minecraftdiamondsword for big CNC schetch rotated_v3 (Autodesk Fusion 360 design; units mm, degrees)
Autodesk Fusion 360 part; units mm, degrees
sketch "big huge diamond sword" plane through (0, 0, 0) normal (0, 0, 1) x (1, 0, 0)
  line L0 (0, 45.2548) -> (5.6569, 39.598)
  line L1 (5.6569, 39.598) -> (11.3137, 45.2548)
  line L2 (11.3137, 45.2548) -> (5.6569, 50.9117)
  line L3 (5.6569, 50.9117) -> (0, 45.2548)
  line L4 (5.6569, 39.598) -> (11.3137, 33.9411)
  line L5 (11.3137, 33.9411) -> (16.9706, 39.598)
  line L6 (16.9706, 39.598) -> (11.3137, 45.2548)
  line L7 (11.3137, 45.2548) -> (5.6569, 39.598)
  line L8 (11.3137, 33.9411) -> (16.9706, 28.2843)
  line L9 (16.9706, 28.2843) -> (22.6274, 33.9411)
  line L10 (16.9706, 39.598) -> (11.3137, 33.9411)
  line L11 (5.6569, 50.9117) -> (11.3137, 45.2548)
  line L12 (11.3137, 45.2548) -> (16.9706, 50.9117)
  line L13 (16.9706, 50.9117) -> (11.3137, 56.5685)
  line L14 (11.3137, 56.5685) -> (5.6569, 50.9117)
  line L15 (16.9706, 50.9117) -> (22.6274, 45.2548)
  line L16 (22.6274, 45.2548) -> (16.9706, 39.598)
  line L17 (16.9706, 39.598) -> (11.3137, 45.2548)
  line L18 (11.3137, 45.2548) -> (16.9706, 50.9117)
  line L19 (11.3137, 56.5685) -> (16.9706, 50.9117)
  line L20 (16.9706, 50.9117) -> (22.6274, 56.5685)
  line L21 (22.6274, 56.5685) -> (16.9706, 62.2254)
  line L22 (16.9706, 62.2254) -> (11.3137, 56.5685)
  line L23 (16.9706, 50.9117) -> (22.6274, 45.2548)
  line L24 (22.6274, 45.2548) -> (28.2843, 50.9117)
  line L25 (28.2843, 50.9117) -> (22.6274, 56.5685)
  line L26 (22.6274, 56.5685) -> (16.9706, 50.9117)
  line L27 (22.6274, 45.2548) -> (28.2843, 39.598)
  line L28 (28.2843, 39.598) -> (22.6274, 33.9411)
  line L29 (22.6274, 33.9411) -> (16.9706, 39.598)
  line L30 (16.9706, 39.598) -> (22.6274, 45.2548)
  line L31 (22.6274, 45.2548) -> (28.2843, 39.598)
  line L32 (28.2843, 39.598) -> (33.9411, 45.2548)
  line L33 (33.9411, 45.2548) -> (28.2843, 50.9117)
  line L34 (28.2843, 50.9117) -> (22.6274, 45.2548)
  line L35 (28.2843, 50.9117) -> (33.9411, 45.2548)
  line L36 (33.9411, 45.2548) -> (39.598, 50.9117)
  line L37 (39.598, 50.9117) -> (33.9411, 56.5685)
  line L38 (33.9411, 56.5685) -> (28.2843, 50.9117)
  line L39 (33.9411, 45.2548) -> (39.598, 39.598)
  line L40 (39.598, 39.598) -> (33.9411, 33.9411)
  line L41 (33.9411, 33.9411) -> (28.2843, 39.598)
  line L42 (28.2843, 39.598) -> (33.9411, 45.2548)
  line L43 (33.9411, 45.2548) -> (39.598, 39.598)
  line L44 (39.598, 39.598) -> (45.2548, 45.2548)
  line L45 (45.2548, 45.2548) -> (39.598, 50.9117)
  line L46 (39.598, 50.9117) -> (33.9411, 45.2548)
  line L47 (39.598, 50.9117) -> (45.2548, 45.2548)
  line L48 (45.2548, 45.2548) -> (50.9117, 50.9117)
  line L49 (50.9117, 50.9117) -> (45.2548, 56.5685)
  line L50 (45.2548, 56.5685) -> (39.598, 50.9117)
  line L51 (45.2548, 45.2548) -> (50.9117, 39.598)
  line L52 (45.2548, 33.9411) -> (39.598, 39.598)
  line L53 (39.598, 39.598) -> (45.2548, 45.2548)
  line L54 (45.2548, 45.2548) -> (50.9117, 39.598)
  line L55 (50.9117, 39.598) -> (56.5685, 45.2548)
  line L56 (56.5685, 45.2548) -> (50.9117, 50.9117)
  line L57 (50.9117, 50.9117) -> (45.2548, 45.2548)
  line L58 (50.9117, 50.9117) -> (56.5685, 45.2548)
  line L59 (56.5685, 45.2548) -> (62.2254, 50.9117)
  line L60 (62.2254, 50.9117) -> (56.5685, 56.5685)
  line L61 (56.5685, 56.5685) -> (50.9117, 50.9117)
  line L62 (56.5685, 56.5685) -> (50.9117, 62.2254)
  line L63 (50.9117, 62.2254) -> (56.5685, 67.8823)
  line L64 (56.5685, 67.8823) -> (62.2254, 62.2254)
  line L65 (62.2254, 62.2254) -> (56.5685, 56.5685)
  line L66 (56.5685, 67.8823) -> (62.2254, 62.2254)
  line L67 (62.2254, 62.2254) -> (67.8823, 67.8823)
  line L68 (67.8823, 67.8823) -> (62.2254, 73.5391)
  line L69 (62.2254, 73.5391) -> (56.5685, 67.8823)
  line L70 (62.2254, 73.5391) -> (56.5685, 79.196)
  line L71 (56.5685, 79.196) -> (62.2254, 84.8528)
  line L72 (62.2254, 84.8528) -> (67.8823, 79.196)
  line L73 (67.8823, 79.196) -> (62.2254, 73.5391)
  line L74 (62.2254, 84.8528) -> (67.8823, 79.196)
  line L75 (67.8823, 79.196) -> (73.5391, 84.8528)
  line L76 (73.5391, 84.8528) -> (67.8823, 90.5097)
  line L77 (67.8823, 90.5097) -> (62.2254, 84.8528)
  line L78 (67.8823, 79.196) -> (73.5391, 73.5391)
  line L79 (73.5391, 73.5391) -> (79.196, 79.196)
  line L80 (79.196, 79.196) -> (73.5391, 84.8528)
  line L81 (73.5391, 84.8528) -> (67.8823, 79.196)
  line L82 (62.2254, 73.5391) -> (67.8823, 67.8823)
  line L83 (67.8823, 67.8823) -> (73.5391, 73.5391)
  line L84 (73.5391, 73.5391) -> (67.8823, 79.196)
  line L85 (67.8823, 79.196) -> (62.2254, 73.5391)
  line L86 (73.5391, 73.5391) -> (79.196, 67.8823)
  line L87 (79.196, 67.8823) -> (73.5391, 62.2254)
  line L88 (73.5391, 62.2254) -> (67.8823, 67.8823)
  line L89 (67.8823, 67.8823) -> (73.5391, 73.5391)
  line L90 (67.8823, 67.8823) -> (73.5391, 62.2254)
  line L91 (73.5391, 62.2254) -> (67.8823, 56.5685)
  line L92 (67.8823, 56.5685) -> (62.2254, 62.2254)
  line L93 (62.2254, 62.2254) -> (67.8823, 67.8823)
  line L94 (56.5685, 56.5685) -> (62.2254, 50.9117)
  line L95 (62.2254, 50.9117) -> (67.8823, 56.5685)
  line L96 (67.8823, 56.5685) -> (62.2254, 62.2254)
  line L97 (62.2254, 62.2254) -> (56.5685, 56.5685)
  line L98 (50.9117, 39.598) -> (56.5685, 33.9411)
  line L99 (45.2548, 33.9411) -> (50.9117, 39.598)
  line L100 (56.5685, 45.2548) -> (62.2254, 39.598)
  line L101 (62.2254, 39.598) -> (56.5685, 33.9411)
  line L102 (50.9117, 39.598) -> (56.5685, 45.2548)
  line L103 (62.2254, 50.9117) -> (67.8823, 45.2548)
  line L104 (67.8823, 45.2548) -> (62.2254, 39.598)
  line L105 (62.2254, 39.598) -> (56.5685, 45.2548)
  line L106 (56.5685, 45.2548) -> (62.2254, 50.9117)
  line L107 (56.5685, 33.9411) -> (62.2254, 28.2843)
  line L108 (62.2254, 28.2843) -> (56.5685, 22.6274)
  line L109 (56.5685, 22.6274) -> (50.9117, 28.2843)
  line L110 (50.9117, 28.2843) -> (56.5685, 33.9411)
  line L111 (56.5685, 33.9411) -> (62.2254, 28.2843)
  line L112 (62.2254, 28.2843) -> (67.8823, 33.9411)
  line L113 (67.8823, 33.9411) -> (62.2254, 39.598)
  line L114 (62.2254, 39.598) -> (56.5685, 33.9411)
  line L115 (62.2254, 28.2843) -> (67.8823, 22.6274)
  line L116 (67.8823, 22.6274) -> (62.2254, 16.9706)
  line L117 (62.2254, 16.9706) -> (56.5685, 22.6274)
  line L118 (56.5685, 22.6274) -> (62.2254, 28.2843)
  line L119 (62.2254, 16.9706) -> (67.8823, 11.3137)
  line L120 (67.8823, 11.3137) -> (73.5391, 16.9706)
  line L121 (73.5391, 16.9706) -> (67.8823, 22.6274)
  line L122 (67.8823, 22.6274) -> (62.2254, 16.9706)
  line L123 (67.8823, 11.3137) -> (73.5391, 5.6569)
  line L124 (73.5391, 5.6569) -> (79.196, 11.3137)
  line L125 (79.196, 11.3137) -> (73.5391, 16.9706)
  line L126 (73.5391, 16.9706) -> (67.8823, 11.3137)
  line L127 (62.2254, 16.9706) -> (67.8823, 11.3137)
  line L128 (67.8823, 11.3137) -> (62.2254, 5.6569)
  line L129 (62.2254, 5.6569) -> (56.5685, 11.3137)
  line L130 (56.5685, 11.3137) -> (62.2254, 16.9706)
  line L131 (67.8823, 11.3137) -> (73.5391, 5.6569)
  line L132 (73.5391, 5.6569) -> (67.8823, 0)
  line L133 (67.8823, 0) -> (62.2254, 5.6569)
  line L134 (62.2254, 5.6569) -> (67.8823, 11.3137)
  line L135 (67.8823, 56.5685) -> (73.5391, 50.9117)
  line L136 (73.5391, 50.9117) -> (67.8823, 45.2548)
  line L137 (67.8823, 45.2548) -> (62.2254, 50.9117)
  line L138 (62.2254, 50.9117) -> (67.8823, 56.5685)
  line L139 (67.8823, 45.2548) -> (73.5391, 39.598)
  line L140 (73.5391, 39.598) -> (67.8823, 33.9411)
  line L141 (67.8823, 33.9411) -> (62.2254, 39.598)
  line L142 (62.2254, 39.598) -> (67.8823, 45.2548)
  line L143 (73.5391, 62.2254) -> (79.196, 56.5685)
  line L144 (79.196, 56.5685) -> (73.5391, 50.9117)
  line L145 (73.5391, 50.9117) -> (67.8823, 56.5685)
  line L146 (67.8823, 56.5685) -> (73.5391, 62.2254)
  line L147 (73.5391, 50.9117) -> (79.196, 45.2548)
  line L148 (79.196, 45.2548) -> (73.5391, 39.598)
  line L149 (73.5391, 39.598) -> (67.8823, 45.2548)
  line L150 (67.8823, 45.2548) -> (73.5391, 50.9117)
  line L151 (79.196, 56.5685) -> (84.8528, 50.9117)
  line L152 (84.8528, 50.9117) -> (79.196, 45.2548)
  line L153 (79.196, 45.2548) -> (73.5391, 50.9117)
  line L154 (73.5391, 50.9117) -> (79.196, 56.5685)
  line L155 (67.8823, 33.9411) -> (73.5391, 28.2843)
  line L156 (73.5391, 28.2843) -> (67.8823, 22.6274)
  line L157 (67.8823, 22.6274) -> (62.2254, 28.2843)
  line L158 (62.2254, 28.2843) -> (67.8823, 33.9411)
  line L159 (73.5391, 28.2843) -> (79.196, 22.6274)
  line L160 (79.196, 22.6274) -> (73.5391, 16.9706)
  line L161 (73.5391, 16.9706) -> (67.8823, 22.6274)
  line L162 (67.8823, 22.6274) -> (73.5391, 28.2843)
  line L163 (73.5391, 39.598) -> (79.196, 33.9411)
  line L164 (79.196, 33.9411) -> (73.5391, 28.2843)
  line L165 (73.5391, 28.2843) -> (67.8823, 33.9411)
  line L166 (67.8823, 33.9411) -> (73.5391, 39.598)
  line L167 (79.196, 45.2548) -> (84.8528, 39.598)
  line L168 (84.8528, 39.598) -> (79.196, 33.9411)
  line L169 (79.196, 33.9411) -> (73.5391, 39.598)
  line L170 (73.5391, 39.598) -> (79.196, 45.2548)
  line L171 (79.196, 33.9411) -> (73.5391, 39.598)
  line L172 (73.5391, 39.598) -> (79.196, 45.2548)
  line L173 (79.196, 45.2548) -> (84.8528, 39.598)
  line L174 (84.8528, 39.598) -> (79.196, 33.9411)
  line L175 (79.196, 33.9411) -> (84.8528, 28.2843)
  line L176 (84.8528, 28.2843) -> (90.5097, 33.9411)
  line L177 (90.5097, 33.9411) -> (84.8528, 39.598)
  line L178 (84.8528, 39.598) -> (79.196, 33.9411)
  line L179 (79.196, 45.2548) -> (84.8528, 39.598)
  line L180 (84.8528, 39.598) -> (90.5097, 45.2548)
  line L181 (90.5097, 45.2548) -> (84.8528, 50.9117)
  line L182 (84.8528, 50.9117) -> (79.196, 45.2548)
  line L183 (84.8528, 39.598) -> (90.5097, 33.9411)
  line L184 (90.5097, 33.9411) -> (96.1665, 39.598)
  line L185 (96.1665, 39.598) -> (90.5097, 45.2548)
  line L186 (90.5097, 45.2548) -> (84.8528, 39.598)
  line L187 (90.5097, 33.9411) -> (96.1665, 28.2843)
  line L188 (96.1665, 28.2843) -> (101.8234, 33.9411)
  line L189 (101.8234, 33.9411) -> (96.1665, 39.598)
  line L190 (96.1665, 39.598) -> (90.5097, 33.9411)
  line L191 (79.196, 56.5685) -> (84.8528, 50.9117)
  line L192 (84.8528, 50.9117) -> (90.5097, 56.5685)
  line L193 (90.5097, 56.5685) -> (84.8528, 62.2254)
  line L194 (84.8528, 62.2254) -> (79.196, 56.5685)
  line L195 (84.8528, 50.9117) -> (90.5097, 45.2548)
  line L196 (90.5097, 45.2548) -> (96.1665, 50.9117)
  line L197 (96.1665, 50.9117) -> (90.5097, 56.5685)
  line L198 (90.5097, 56.5685) -> (84.8528, 50.9117)
  line L199 (96.1665, 50.9117) -> (90.5097, 56.5685)
  line L200 (90.5097, 56.5685) -> (96.1665, 62.2254)
  line L201 (96.1665, 62.2254) -> (101.8234, 56.5685)
  line L202 (101.8234, 56.5685) -> (96.1665, 50.9117)
  line L203 (90.5097, 45.2548) -> (96.1665, 39.598)
  line L204 (96.1665, 39.598) -> (101.8234, 45.2548)
  line L205 (101.8234, 45.2548) -> (96.1665, 50.9117)
  line L206 (96.1665, 50.9117) -> (90.5097, 45.2548)
  line L207 (96.1665, 50.9117) -> (101.8234, 45.2548)
  line L208 (101.8234, 45.2548) -> (107.4802, 50.9117)
  line L209 (107.4802, 50.9117) -> (101.8234, 56.5685)
  line L210 (101.8234, 56.5685) -> (96.1665, 50.9117)
  line L211 (96.1665, 39.598) -> (101.8234, 33.9411)
  line L212 (101.8234, 33.9411) -> (107.4802, 39.598)
  line L213 (107.4802, 39.598) -> (101.8234, 45.2548)
  line L214 (101.8234, 45.2548) -> (96.1665, 39.598)
  line L215 (101.8234, 56.5685) -> (107.4802, 50.9117)
  line L216 (107.4802, 50.9117) -> (113.1371, 56.5685)
  line L217 (113.1371, 56.5685) -> (107.4802, 62.2254)
  line L218 (107.4802, 62.2254) -> (101.8234, 56.5685)
  line L219 (101.8234, 33.9411) -> (107.4802, 28.2843)
  line L220 (107.4802, 28.2843) -> (113.1371, 33.9411)
  line L221 (113.1371, 33.9411) -> (107.4802, 39.598)
  line L222 (107.4802, 39.598) -> (101.8234, 33.9411)
  line L223 (101.8234, 45.2548) -> (107.4802, 39.598)
  line L224 (107.4802, 39.598) -> (113.1371, 45.2548)
  line L225 (113.1371, 45.2548) -> (107.4802, 50.9117)
  line L226 (107.4802, 50.9117) -> (101.8234, 45.2548)
  line L227 (113.1371, 45.2548) -> (118.7939, 39.598)
  line L228 (118.7939, 39.598) -> (124.4508, 45.2548)
  line L229 (124.4508, 45.2548) -> (118.7939, 50.9117)
  line L230 (118.7939, 50.9117) -> (113.1371, 45.2548)
  line L231 (113.1371, 45.2548) -> (107.4802, 50.9117)
  line L232 (107.4802, 50.9117) -> (113.1371, 56.5685)
  line L233 (113.1371, 56.5685) -> (118.7939, 50.9117)
  line L234 (118.7939, 50.9117) -> (113.1371, 45.2548)
  line L235 (113.1371, 45.2548) -> (118.7939, 39.598)
  line L236 (118.7939, 39.598) -> (113.1371, 33.9411)
  line L237 (113.1371, 33.9411) -> (107.4802, 39.598)
  line L238 (107.4802, 39.598) -> (113.1371, 45.2548)
  line L239 (113.1371, 56.5685) -> (118.7939, 50.9117)
  line L240 (118.7939, 50.9117) -> (124.4508, 56.5685)
  line L241 (124.4508, 56.5685) -> (118.7939, 62.2254)
  line L242 (118.7939, 62.2254) -> (113.1371, 56.5685)
  line L243 (118.7939, 50.9117) -> (124.4508, 45.2548)
  line L244 (124.4508, 45.2548) -> (130.1076, 50.9117)
  line L245 (130.1076, 50.9117) -> (124.4508, 56.5685)
  line L246 (124.4508, 56.5685) -> (118.7939, 50.9117)
  line L247 (113.1371, 33.9411) -> (118.7939, 28.2843)
  line L248 (118.7939, 28.2843) -> (124.4508, 33.9411)
  line L249 (124.4508, 33.9411) -> (118.7939, 39.598)
  line L250 (118.7939, 39.598) -> (113.1371, 33.9411)
  line L251 (118.7939, 39.598) -> (124.4508, 33.9411)
  line L252 (124.4508, 33.9411) -> (130.1076, 39.598)
  line L253 (130.1076, 39.598) -> (124.4508, 45.2548)
  line L254 (124.4508, 45.2548) -> (118.7939, 39.598)
  line L255 (124.4508, 45.2548) -> (130.1076, 39.598)
  line L256 (130.1076, 39.598) -> (135.7645, 45.2548)
  line L257 (135.7645, 45.2548) -> (130.1076, 50.9117)
  line L258 (130.1076, 50.9117) -> (124.4508, 45.2548)
  line L259 (124.4508, 56.5685) -> (130.1076, 50.9117)
  line L260 (130.1076, 50.9117) -> (135.7645, 56.5685)
  line L261 (135.7645, 56.5685) -> (130.1076, 62.2254)
  line L262 (130.1076, 62.2254) -> (124.4508, 56.5685)
  line L263 (124.4508, 33.9411) -> (130.1076, 28.2843)
  line L264 (130.1076, 28.2843) -> (135.7645, 33.9411)
  line L265 (135.7645, 33.9411) -> (130.1076, 39.598)
  line L266 (130.1076, 39.598) -> (124.4508, 33.9411)
  line L267 (130.1076, 50.9117) -> (135.7645, 45.2548)
  line L268 (135.7645, 45.2548) -> (141.4214, 50.9117)
  line L269 (141.4214, 50.9117) -> (135.7645, 56.5685)
  line L270 (135.7645, 56.5685) -> (130.1076, 50.9117)
  line L271 (130.1076, 39.598) -> (135.7645, 33.9411)
  line L272 (135.7645, 33.9411) -> (141.4214, 39.598)
  line L273 (141.4214, 39.598) -> (135.7645, 45.2548)
  line L274 (135.7645, 45.2548) -> (130.1076, 39.598)
  line L275 (135.7645, 45.2548) -> (141.4214, 39.598)
  line L276 (141.4214, 39.598) -> (147.0782, 45.2548)
  line L277 (147.0782, 45.2548) -> (141.4214, 50.9117)
  line L278 (141.4214, 50.9117) -> (135.7645, 45.2548)
  line L279 (135.7645, 33.9411) -> (141.4214, 28.2843)
  line L280 (141.4214, 28.2843) -> (147.0782, 33.9411)
  line L281 (147.0782, 33.9411) -> (141.4214, 39.598)
  line L282 (141.4214, 39.598) -> (135.7645, 33.9411)
  line L283 (135.7645, 56.5685) -> (141.4214, 50.9117)
  line L284 (141.4214, 50.9117) -> (147.0782, 56.5685)
  line L285 (147.0782, 56.5685) -> (141.4214, 62.2254)
  line L286 (141.4214, 62.2254) -> (135.7645, 56.5685)
  line L287 (147.0782, 45.2548) -> (152.7351, 39.598)
  line L288 (152.7351, 39.598) -> (147.0782, 33.9411)
  line L289 (147.0782, 33.9411) -> (141.4214, 39.598)
  line L290 (141.4214, 39.598) -> (147.0782, 45.2548)
  line L291 (141.4214, 50.9117) -> (147.0782, 45.2548)
  line L292 (147.0782, 45.2548) -> (152.7351, 50.9117)
  line L293 (152.7351, 50.9117) -> (147.0782, 56.5685)
  line L294 (147.0782, 56.5685) -> (141.4214, 50.9117)
  line L295 (147.0782, 45.2548) -> (152.7351, 39.598)
  line L296 (152.7351, 39.598) -> (158.3919, 45.2548)
  line L297 (158.3919, 45.2548) -> (152.7351, 50.9117)
  line L298 (152.7351, 50.9117) -> (147.0782, 45.2548)
  line L299 (147.0782, 33.9411) -> (152.7351, 28.2843)
  line L300 (152.7351, 28.2843) -> (158.3919, 33.9411)
  line L301 (158.3919, 33.9411) -> (152.7351, 39.598)
  line L302 (152.7351, 39.598) -> (147.0782, 33.9411)
  line L303 (147.0782, 56.5685) -> (152.7351, 50.9117)
  line L304 (152.7351, 50.9117) -> (158.3919, 56.5685)
  line L305 (158.3919, 56.5685) -> (152.7351, 62.2254)
  line L306 (152.7351, 62.2254) -> (147.0782, 56.5685)
  line L307 (158.3919, 56.5685) -> (164.0488, 50.9117)
  line L308 (164.0488, 50.9117) -> (158.3919, 45.2548)
  line L309 (158.3919, 45.2548) -> (152.7351, 50.9117)
  line L310 (152.7351, 50.9117) -> (158.3919, 56.5685)
  line L311 (152.7351, 39.598) -> (158.3919, 33.9411)
  line L312 (158.3919, 33.9411) -> (164.0488, 39.598)
  line L313 (164.0488, 39.598) -> (158.3919, 45.2548)
  line L314 (158.3919, 45.2548) -> (152.7351, 39.598)
  line L315 (158.3919, 45.2548) -> (164.0488, 39.598)
  line L316 (164.0488, 39.598) -> (169.7056, 45.2548)
  line L317 (169.7056, 45.2548) -> (164.0488, 50.9117)
  line L318 (164.0488, 50.9117) -> (158.3919, 45.2548)
  line L319 (158.3919, 56.5685) -> (164.0488, 50.9117)
  line L320 (164.0488, 50.9117) -> (169.7056, 56.5685)
  line L321 (169.7056, 56.5685) -> (164.0488, 62.2254)
  line L322 (164.0488, 62.2254) -> (158.3919, 56.5685)
  line L323 (164.0488, 50.9117) -> (169.7056, 45.2548)
  line L324 (169.7056, 45.2548) -> (175.3625, 50.9117)
  line L325 (175.3625, 50.9117) -> (169.7056, 56.5685)
  line L326 (169.7056, 56.5685) -> (164.0488, 50.9117)
  line L327 (158.3919, 33.9411) -> (164.0488, 28.2843)
  line L328 (164.0488, 28.2843) -> (169.7056, 33.9411)
  line L329 (169.7056, 33.9411) -> (164.0488, 39.598)
  line L330 (164.0488, 39.598) -> (158.3919, 33.9411)
  line L331 (164.0488, 39.598) -> (169.7056, 33.9411)
  line L332 (169.7056, 33.9411) -> (175.3625, 39.598)
  line L333 (175.3625, 39.598) -> (169.7056, 45.2548)
  line L334 (169.7056, 45.2548) -> (164.0488, 39.598)
  line L335 (169.7056, 45.2548) -> (164.0488, 50.9117)
  line L336 (164.0488, 50.9117) -> (169.7056, 56.5685)
  line L337 (169.7056, 56.5685) -> (175.3625, 50.9117)
  line L338 (175.3625, 50.9117) -> (169.7056, 45.2548)
  line L339 (169.7056, 45.2548) -> (175.3625, 39.598)
  line L340 (175.3625, 39.598) -> (181.0193, 45.2548)
  line L341 (181.0193, 45.2548) -> (175.3625, 50.9117)
  line L342 (175.3625, 50.9117) -> (169.7056, 45.2548)
  dimension "d249" = 8
  dimension "d250" = 8
  dimension "d251" = 8
  dimension "d252" = 8
  dimension "d253" = 8
  dimension "d254" = 8
  dimension "d255" = 8
  dimension "d256" = 8
  dimension "d261" = 8
  dimension "d262" = 8
  dimension "d263" = 8
  dimension "d264" = 8
  dimension "d265" = 8
  dimension "d266" = 8
  dimension "d267" = 8
  dimension "d268" = 8
  dimension "d271" = 8
  dimension "d272" = 8
  dimension "d273" = 8
  dimension "d274" = 8
  dimension "d275" = 8
  dimension "d276" = 8
  dimension "d277" = 8
  dimension "d278" = 8
  dimension "d279" = 8
  dimension "d280" = 8
  dimension "d281" = 8
  dimension "d282" = 8
  dimension "d283" = 8
  dimension "d284" = 8
  dimension "d285" = 8
  dimension "d286" = 8
  dimension "d287" = 8
  dimension "d288" = 8
  dimension "d289" = 8
  dimension "d290" = 8
  dimension "d291" = 8
  dimension "d292" = 8
  dimension "d293" = 8
  dimension "d294" = 8
  dimension "d295" = 8
  dimension "d296" = 8
  dimension "d297" = 8
  dimension "d298" = 8
  dimension "d299" = 8
  dimension "d300" = 8
  dimension "d301" = 8
  dimension "d302" = 8
  dimension "d303" = 8
  dimension "d304" = 8
  dimension "d309" = 8
  dimension "d310" = 8
  dimension "d311" = 8
  dimension "d312" = 8
  dimension "d313" = 8
  dimension "d314" = 8
  dimension "d315" = 8
  dimension "d316" = 8
  dimension "d319" = 8
  dimension "d320" = 8
  dimension "d321" = 8
  dimension "d322" = 8
  dimension "d323" = 8
  dimension "d324" = 8
  dimension "d325" = 8
  dimension "d326" = 8
  dimension "d327" = 8
  dimension "d328" = 8
  dimension "d329" = 8
  dimension "d330" = 8
  dimension "d331" = 8
  dimension "d332" = 8
  dimension "d333" = 8
  dimension "d334" = 8
  dimension "d335" = 8
  dimension "d336" = 8
  dimension "d337" = 8
  dimension "d338" = 8
  dimension "d339" = 8
  dimension "d340" = 8
  dimension "d341" = 8
  dimension "d342" = 8
  dimension "d343" = 8
  dimension "d344" = 8
  dimension "d345" = 8
  dimension "d346" = 8
  dimension "d347" = 8
  dimension "d348" = 8
  dimension "d349" = 8
  dimension "d350" = 8
  dimension "d351" = 8
  dimension "d352" = 8
  dimension "d353" = 8
  dimension "d354" = 8
  dimension "d355" = 8
  dimension "d356" = 8
  dimension "d357" = 8
  dimension "d358" = 8
  dimension "d359" = 8
  dimension "d360" = 8
  dimension "d361" = 8
  dimension "d362" = 8
  dimension "d363" = 8
  dimension "d364" = 8
  dimension "d365" = 8
  dimension "d366" = 8
  dimension "d367" = 8
  dimension "d368" = 8
  dimension "d369" = 8
  dimension "d370" = 8
  dimension "d371" = 8
  dimension "d372" = 8
  dimension "d373" = 8
  dimension "d374" = 8
  dimension "d375" = 8
  dimension "d376" = 8
  dimension "d377" = 8
  dimension "d378" = 8
  dimension "d379" = 8
  dimension "d380" = 8
  dimension "d381" = 8
  dimension "d382" = 8
  dimension "d383" = 8
  dimension "d384" = 8
  dimension "d385" = 8
  dimension "d386" = 8
  dimension "d387" = 8
  dimension "d388" = 8
  dimension "d389" = 8
  dimension "d390" = 8
  dimension "d391" = 8
  dimension "d392" = 8
  dimension "d393" = 8
  dimension "d394" = 8
  dimension "d395" = 8
  dimension "d396" = 8
  dimension "d397" = 8
  dimension "d398" = 8
  dimension "d399" = 8
  dimension "d400" = 8
  dimension "d401" = 8
  dimension "d402" = 8
  dimension "d403" = 8
  dimension "d404" = 8
  dimension "d405" = 8
  dimension "d406" = 8
  dimension "d407" = 8
  dimension "d408" = 8
  dimension "d409" = 8
  dimension "d410" = 8
  dimension "d411" = 8
  dimension "d412" = 8
  dimension "d413" = 8
  dimension "d414" = 8
  dimension "d415" = 8
  dimension "d416" = 8
  dimension "d417" = 8
  dimension "d418" = 8
  dimension "d419" = 8
  dimension "d420" = 8
  dimension "d421" = 8
  dimension "d422" = 8
  dimension "d423" = 8
  dimension "d424" = 8
  dimension "d425" = 8
  dimension "d426" = 8
  dimension "d427" = 8
  dimension "d428" = 8
  dimension "d429" = 8
  dimension "d430" = 8
  dimension "d431" = 8
  dimension "d432" = 8
  dimension "d433" = 8
  dimension "d434" = 8
  constraint perpendicular L74 L75
  constraint parallel L75 L77
  constraint perpendicular L78 L79
  constraint parallel L79 L81
  constraint perpendicular L86 L87
  constraint parallel L87 L89
  constraint perpendicular L103 L104
  constraint parallel L104 L106
  constraint perpendicular L52 L99
  constraint coincident L98.end L101.end
  constraint perpendicular L115 L116
  constraint parallel L116 L118
  constraint perpendicular L123 L124
  constraint parallel L124 L126
  constraint perpendicular L127 L128
  constraint parallel L128 L130
  constraint perpendicular L131 L132
  constraint parallel L132 L134
  constraint perpendicular L135 L136
  constraint parallel L136 L138
  constraint perpendicular L139 L140
  constraint parallel L140 L142
  constraint perpendicular L143 L144
  constraint parallel L144 L146
  constraint perpendicular L147 L148
  constraint parallel L148 L150
  constraint perpendicular L151 L152
  constraint parallel L152 L154
  constraint perpendicular L155 L156
  constraint parallel L156 L158
  constraint perpendicular L159 L160
  constraint parallel L160 L162
  constraint perpendicular L163 L164
  constraint parallel L164 L166
  constraint perpendicular L167 L168
  constraint parallel L168 L170
  constraint perpendicular L171 L172
  constraint parallel L172 L174
  constraint perpendicular L175 L176
  constraint parallel L176 L178
  constraint perpendicular L179 L180
  constraint parallel L180 L182
  constraint perpendicular L183 L184
  constraint parallel L184 L186
  constraint perpendicular L187 L188
  constraint parallel L188 L190
  constraint perpendicular L195 L196
  constraint parallel L196 L198
  constraint perpendicular L199 L200
  constraint parallel L200 L202
  constraint perpendicular L203 L204
  constraint parallel L204 L206
  constraint perpendicular L211 L212
  constraint parallel L212 L214
  constraint perpendicular L215 L216
  constraint parallel L216 L218
  constraint perpendicular L219 L220
  constraint parallel L220 L222
  constraint perpendicular L223 L224
  constraint parallel L224 L226
  constraint perpendicular L227 L228
  constraint parallel L228 L230
  constraint perpendicular L231 L232
  constraint parallel L232 L234
  constraint perpendicular L235 L236
  constraint parallel L236 L238
  constraint perpendicular L239 L240
  constraint parallel L240 L242
  constraint perpendicular L243 L244
  constraint parallel L244 L246
  constraint perpendicular L247 L248
  constraint parallel L248 L250
  constraint perpendicular L251 L252
  constraint parallel L252 L254
  constraint perpendicular L255 L256
  constraint parallel L256 L258
  constraint perpendicular L259 L260
  constraint parallel L260 L262
  constraint perpendicular L263 L264
  constraint parallel L264 L266
  constraint perpendicular L267 L268
  constraint parallel L268 L270
  constraint perpendicular L275 L276
  constraint parallel L276 L278
  constraint perpendicular L279 L280
  constraint parallel L280 L282
  constraint perpendicular L283 L284
  constraint parallel L284 L286
  constraint perpendicular L287 L288
  constraint parallel L288 L290
  constraint perpendicular L291 L292
  constraint parallel L292 L294
  constraint perpendicular L303 L304
  constraint parallel L304 L306
  constraint perpendicular L339 L340
  constraint parallel L340 L342
  measures "d249" distance of L0.start L0.end
  measures "d250" distance of L0.start L2.end
  measures "d251" distance of L0.end L4.end
  measures "d252" distance of L0.end L1.end
  measures "d253" distance of L4.end L8.end
  measures "d254" distance of L4.end L5.end
  measures "d255" distance of L2.end L1.end
  measures "d256" distance of L2.end L13.end
  measures "d261" distance of L12.end L15.end
  measures "d262" distance of L12.end L1.end
  measures "d263" distance of L13.end L12.end
  measures "d264" distance of L13.end L21.end
  measures "d265" distance of L12.end L15.end
  measures "d266" distance of L12.end L20.end
  measures "d267" distance of L15.end L27.end
  measures "d268" distance of L15.end L5.end
  measures "d271" distance of L15.end L27.end
  measures "d272" distance of L15.end L24.end
  measures "d273" distance of L24.end L32.end
  measures "d274" distance of L24.end L37.end
  measures "d275" distance of L32.end L39.end
  measures "d276" distance of L32.end L27.end
  measures "d277" distance of L32.end L39.end
  measures "d278" distance of L32.end L36.end
  measures "d279" distance of L36.end L44.end
  measures "d280" distance of L36.end L49.end
  measures "d281" distance of L44.end L51.end
  measures "d282" distance of L44.end L39.end
  measures "d283" distance of L44.end L51.end
  measures "d284" distance of L44.end L48.end
  measures "d285" distance of L48.end L55.end
  measures "d286" distance of L48.end L60.end
  measures "d287" distance of L60.end L62.end
  measures "d288" distance of L60.end L64.end
  measures "d289" distance of L63.end L64.end
  measures "d290" distance of L63.end L68.end
  measures "d291" distance of L68.end L70.end
  measures "d292" distance of L68.end L72.end
  measures "d293" distance of L71.end L72.end
  measures "d294" distance of L71.end L76.end
  measures "d295" distance of L72.end L78.end
  measures "d296" distance of L72.end L75.end
  measures "d297" distance of L68.end L67.end
  measures "d298" distance of L68.end L72.end
  measures "d299" distance of L78.end L86.end
  measures "d300" distance of L78.end L67.end
  measures "d301" distance of L67.end L87.end
  measures "d302" distance of L67.end L64.end
  measures "d303" distance of L60.end L59.end
  measures "d304" distance of L60.end L64.end
  measures "d309" distance of L51.end L98.end
  measures "d310" distance of L51.end L52.start
  measures "d311" distance of L55.end L100.end
  measures "d312" distance of L55.end L51.end
  measures "d313" distance of L59.end L103.end
  measures "d314" distance of L59.end L55.end
  measures "d315" distance of L98.end L107.end
  measures "d316" distance of L98.end L109.end
  measures "d319" distance of L98.end L107.end
  measures "d320" distance of L98.end L100.end
  measures "d321" distance of L107.end L115.end
  measures "d322" distance of L107.end L108.end
  measures "d323" distance of L116.end L119.end
  measures "d324" distance of L116.end L115.end
  measures "d325" distance of L119.end L123.end
  measures "d326" distance of L119.end L120.end
  measures "d327" distance of L116.end L119.end
  measures "d328" distance of L116.end L129.end
  measures "d329" distance of L119.end L123.end
  measures "d330" distance of L119.end L128.end
  measures "d331" distance of L91.end L135.end
  measures "d332" distance of L91.end L59.end
  measures "d333" distance of L103.end L139.end
  measures "d334" distance of L103.end L100.end
  measures "d335" distance of L87.end L143.end
  measures "d336" distance of L87.end L91.end
  measures "d337" distance of L135.end L147.end
  measures "d338" distance of L135.end L103.end
  measures "d339" distance of L143.end L151.end
  measures "d340" distance of L143.end L135.end
  measures "d341" distance of L112.end L155.end
  measures "d342" distance of L112.end L107.end
  measures "d343" distance of L155.end L159.end
  measures "d344" distance of L155.end L115.end
  measures "d345" distance of L139.end L163.end
  measures "d346" distance of L139.end L112.end
  measures "d347" distance of L147.end L167.end
  measures "d348" distance of L147.end L139.end
  measures "d349" distance of L163.end L139.end
  measures "d350" distance of L163.end L167.end
  measures "d351" distance of L163.end L175.end
  measures "d352" distance of L163.end L167.end
  measures "d353" distance of L147.end L167.end
  measures "d354" distance of L147.end L151.end
  measures "d355" distance of L167.end L176.end
  measures "d356" distance of L167.end L180.end
  measures "d357" distance of L176.end L187.end
  measures "d358" distance of L176.end L184.end
  measures "d359" distance of L143.end L151.end
  measures "d360" distance of L143.end L193.end
  measures "d361" distance of L151.end L180.end
  measures "d362" distance of L151.end L192.end
  measures "d363" distance of L196.end L192.end
  measures "d364" distance of L196.end L201.end
  measures "d365" distance of L180.end L184.end
  measures "d366" distance of L180.end L196.end
  measures "d367" distance of L196.end L204.end
  measures "d368" distance of L196.end L201.end
  measures "d369" distance of L184.end L188.end
  measures "d370" distance of L184.end L204.end
  measures "d371" distance of L201.end L208.end
  measures "d372" distance of L201.end L217.end
  measures "d373" distance of L188.end L219.end
  measures "d374" distance of L188.end L212.end
  measures "d375" distance of L204.end L212.end
  measures "d376" distance of L204.end L208.end
  measures "d377" distance of L224.end L227.end
  measures "d378" distance of L224.end L229.end
  measures "d379" distance of L224.end L208.end
  measures "d380" distance of L224.end L229.end
  measures "d381" distance of L224.end L227.end
  measures "d382" distance of L224.end L212.end
  measures "d383" distance of L216.end L229.end
  measures "d384" distance of L216.end L241.end
  measures "d385" distance of L229.end L228.end
  measures "d386" distance of L229.end L240.end
  measures "d387" distance of L220.end L247.end
  measures "d388" distance of L220.end L227.end
  measures "d389" distance of L227.end L248.end
  measures "d390" distance of L227.end L228.end
  measures "d391" distance of L228.end L252.end
  measures "d392" distance of L228.end L244.end
  measures "d393" distance of L240.end L244.end
  measures "d394" distance of L240.end L261.end
  measures "d395" distance of L248.end L263.end
  measures "d396" distance of L248.end L252.end
  measures "d397" distance of L244.end L256.end
  measures "d398" distance of L244.end L260.end
  measures "d399" distance of L252.end L264.end
  measures "d400" distance of L252.end L256.end
  measures "d401" distance of L256.end L272.end
  measures "d402" distance of L256.end L268.end
  measures "d403" distance of L264.end L279.end
  measures "d404" distance of L264.end L272.end
  measures "d405" distance of L260.end L268.end
  measures "d406" distance of L260.end L285.end
  measures "d407" distance of L276.end L287.end
  measures "d408" distance of L276.end L272.end
  measures "d409" distance of L268.end L276.end
  measures "d410" distance of L268.end L284.end
  measures "d411" distance of L276.end L287.end
  measures "d412" distance of L276.end L292.end
  measures "d413" distance of L280.end L299.end
  measures "d414" distance of L280.end L287.end
  measures "d415" distance of L284.end L292.end
  measures "d416" distance of L284.end L305.end
  measures "d417" distance of L304.end L307.end
  measures "d418" distance of L304.end L292.end
  measures "d419" distance of L287.end L300.end
  measures "d420" distance of L287.end L296.end
  measures "d421" distance of L296.end L312.end
  measures "d422" distance of L296.end L307.end
  measures "d423" distance of L304.end L307.end
  measures "d424" distance of L304.end L321.end
  measures "d425" distance of L307.end L316.end
  measures "d426" distance of L307.end L320.end
  measures "d427" distance of L300.end L327.end
  measures "d428" distance of L300.end L312.end
  measures "d429" distance of L312.end L328.end
  measures "d430" distance of L312.end L316.end
  measures "d431" distance of L316.end L307.end
  measures "d432" distance of L316.end L324.end
  measures "d433" distance of L316.end L332.end
  measures "d434" distance of L316.end L324.end
extrude "Extrude11" add sketch "big huge diamond sword" along normal blind 23 makes body 1
sketch "board prepare" plane through (0, 0, 0) normal (0, 0, 1) x (1, 0, 0)
  line L0 (0, 0) -> (310, 0)
  line L1 (310, 0) -> (310, 124)
  line L2 (310, 124) -> (0, 124)
  line L3 (0, 124) -> (0, 0)
  dimension "d437" = 310
  dimension "d438" = 124
  constraint horizontal L0
  constraint vertical L1
  constraint horizontal L2
  constraint vertical L3
  constraint coincident L0.start L3.end
  measures "d437" distance of L0.start L0.end
  measures "d438" distance of L0.start L2.end
extrude "Extrude12" add sketch "board prepare" along normal blind 23 separate body makes body 2
move_body "Move2" bodies 1 to x (1, 0, 0) y (0, 1, 0) z (0, 0, 1) at (0, 0, 0)
move_body "Move3" bodies 1 to x (1, 0, 0) y (0, 1, 0) z (0, 0, 1) at (136.2, 74.374, -13.1911)
move_body "Move4" bodies 1 to x (1, 0, 0) y (0, 1, 0) z (0, 0, 1) at (-69.7513, -74.374, -19.9999)
move_body "Move5" bodies 1 to x (1, 0, 0) y (0, 1, 0) z (0, 0, 1) at (-66.4487, 7.3542, 0)
move_body "Move6" bodies 1 to x (1, 0, 0) y (0, 1, 0) z (0, 0, 1) at (0, 0, 33.191)
move_body "Move7" bodies 1 to x (1, 0, 0) y (0, 1, 0) z (0, 0, 1) at (-0.0003, -7.3542, 0)
equation "d = 8 mm"
equation "StockHeight = 23 mm"
equation "d249 = d"
equation "d250 = d"
equation "d251 = d"
equation "d252 = d"
equation "d253 = d"
equation "d254 = d"
equation "d255 = d"
equation "d256 = d"
equation "d261 = d"
equation "d262 = d"
equation "d263 = d"
equation "d264 = d"
equation "d265 = d"
equation "d266 = d"
equation "d267 = d"
equation "d268 = d"
equation "d271 = d"
equation "d272 = d"
equation "d273 = d"
equation "d274 = d"
equation "d275 = d"
equation "d276 = d"
equation "d277 = d"
equation "d278 = d"
equation "d279 = d"
equation "d280 = d"
equation "d281 = d"
equation "d282 = d"
equation "d283 = d"
equation "d284 = d"
equation "d285 = d"
equation "d286 = d"
equation "d287 = d"
equation "d288 = d"
equation "d289 = d"
equation "d290 = d"
equation "d291 = d"
equation "d292 = d"
equation "d293 = d"
equation "d294 = d"
equation "d295 = d"
equation "d296 = d"
equation "d297 = d"
equation "d298 = d"
equation "d299 = d"
equation "d300 = d"
equation "d301 = d"
equation "d302 = d"
equation "d303 = d"
equation "d304 = d"
equation "d309 = d"
equation "d310 = d"
equation "d311 = d"
equation "d312 = d"
equation "d313 = d"
equation "d314 = d"
equation "d315 = d"
equation "d316 = d"
equation "d319 = d"
equation "d320 = d"
equation "d321 = d"
equation "d322 = d"
equation "d323 = d"
equation "d324 = d"
equation "d325 = d"
equation "d326 = d"
equation "d327 = d"
equation "d328 = d"
equation "d329 = d"
equation "d330 = d"
equation "d331 = d"
equation "d332 = d"
equation "d333 = d"
equation "d334 = d"
equation "d335 = d"
equation "d336 = d"
equation "d337 = d"
equation "d338 = d"
equation "d339 = d"
equation "d340 = d"
equation "d341 = d"
equation "d342 = d"
equation "d343 = d"
equation "d344 = d"
equation "d345 = d"
equation "d346 = d"
equation "d347 = d"
equation "d348 = d"
equation "d349 = d"
equation "d350 = d"
equation "d351 = d"
equation "d352 = d"
equation "d353 = d"
equation "d354 = d"
equation "d355 = d"
equation "d356 = d"
equation "d357 = d"
equation "d358 = d"
equation "d359 = d"
equation "d360 = d"
equation "d361 = d"
equation "d362 = d"
equation "d363 = d"
equation "d364 = d"
equation "d365 = d"
equation "d366 = d"
equation "d367 = d"
equation "d368 = d"
equation "d369 = d"
equation "d370 = d"
equation "d371 = d"
equation "d372 = d"
equation "d373 = d"
equation "d374 = d"
equation "d375 = d"
equation "d376 = d"
equation "d377 = d"
equation "d378 = d"
equation "d379 = d"
equation "d380 = d"
equation "d381 = d"
equation "d382 = d"
equation "d383 = d"
equation "d384 = d"
equation "d385 = d"
equation "d386 = d"
equation "d387 = d"
equation "d388 = d"
equation "d389 = d"
equation "d390 = d"
equation "d391 = d"
equation "d392 = d"
equation "d393 = d"
equation "d394 = d"
equation "d395 = d"
equation "d396 = d"
equation "d397 = d"
equation "d398 = d"
equation "d399 = d"
equation "d400 = d"
equation "d401 = d"
equation "d402 = d"
equation "d403 = d"
equation "d404 = d"
equation "d405 = d"
equation "d406 = d"
equation "d407 = d"
equation "d408 = d"
equation "d409 = d"
equation "d410 = d"
equation "d411 = d"
equation "d412 = d"
equation "d413 = d"
equation "d414 = d"
equation "d415 = d"
equation "d416 = d"
equation "d417 = d"
equation "d418 = d"
equation "d419 = d"
equation "d420 = d"
equation "d421 = d"
equation "d422 = d"
equation "d423 = d"
equation "d424 = d"
equation "d425 = d"
equation "d426 = d"
equation "d427 = d"
equation "d428 = d"
equation "d429 = d"
equation "d430 = d"
equation "d431 = d"
equation "d432 = d"
equation "d433 = d"
equation "d434 = d"
equation "d435 = StockHeight"
named bodies: "diamond sword body", "board"
